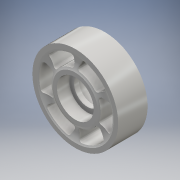
# Autodesk Inventor part: inner_wheel1
Saved by Autodesk Inventor 2016 (Build 200138000, 138)
## iProperties
Created: 2016-02-01
Part Number: inner_wheel1
Material: Aluminum 6061
Document SubType Name: Modeling
Designer: Carlo
Mass: 123.47 g
Surface Area: 198.887 cm^2
Volume: 45.7297 cm^3
Density: 2.7 g/cm^3
Appearance: Aluminum - Flat
Author: Carlo
Autodesk Inventor part; units mm, degrees
ref_plane "YZ Plane" through (0, 0, 0) normal (1, 0, 0) x (0, 1, 0)
ref_plane "XZ Plane" through (0, 0, 0) normal (0, 1, 0) x (-1, 0, 0)
ref_plane "XY Plane" through (0, 0, 0) normal (0, 0, 1) x (1, 0, 0)
sketch "Sketch1" plane through (0, 0, 0) normal (0, 1, 0) x (-1, 0, 0)
  circle A0 centre (0, 0) radius 35
  dimension "d0" = 70
  constraints: 1 centre point, 1 coincident
  measures "d0" diameter of A0
extrude "Extrusion1" add sketch "Sketch1" along normal mid plane 24
sketch "Sketch2" plane through (0, 12, 0) normal (0, 1, 0) x (1, 0, 0)
  line L0 (-24.5746, 17.2073) -> (-16.383, 11.4715)
  line L1 (-5.4819, 29.4949) -> (0, 20)
  arc A0 (-5.4819, 29.4949) -> (-24.5746, 17.2073) centre (0, 0) ccw
  arc A1 (0, 20) -> (-16.383, 11.4715) centre (0, 0) ccw
  line L2 (-16.383, 11.4715) -> (0, 0) construction
  line L3 (0, 0) -> (0, 35) construction
  circle A2 centre (0, 0) radius 35 construction
  dimension "d3" = 30
  dimension "d4" = 55
  dimension "d5" = 30
  dimension "d6" = 20
  constraints: 8 end point, 4 point on circle, 2 centre point, 1 collinear, 1 concentric, 1 point on line, 1 vertical, 1 vertical alignment, 2 other
  measures "d3" angle of L3 L1
  measures "d4" angle of L0 L3
  measures "d5" radius of A0
  measures "d6" radius of A1
extrude "Extrusion2" cut sketch "Sketch2" against normal through all
fillet "Fillet1" radius 2 4 edges at (-24.5746, 0, -17.2073) (-16.383, 0, -11.4715) (0, 0, -20) (-5.4819, 0, -29.4949)
pattern_circular "Circular Pattern1" count 6 over 360 about axis through (0, -10, 0) along (0, 1, 0) of "Extrusion2", "Fillet1"
hole "Hole1" at (0, 12, 0) direction (0, -1, 0) diameter 22 end through all
sketch "Sketch3" plane through (0, 12, 0) normal (0, 1, 0) x (1, 0, 0)
  point P0 (0, 0)
sketch "Sketch4" plane through (0, 12, 0) normal (0, 1, 0) x (1, 0, 0)
  point P0 (0, 0)
sketch "Sketch5" plane through (0, 12, 0) normal (0, 1, 0) x (1, 0, 0)
  circle A0 centre (0, 0) radius 15
  circle A1 centre (0, 0) radius 11 projected
  dimension "d22" = 30
  constraints: 1 centre point, 1 coincident, 1 concentric
  measures "d22" diameter of A0
extrude "Extrusion3" cut sketch "Sketch5" against normal blind 10
sketch "Sketch6" plane through (0, 0, 0) normal (0, 0, 1) x (1, 0, 0)
  line L0 (30, -12) -> (30, 12) projected
  line L1 (30, 12) -> (35, 12) projected
  line L2 (35, 12) -> (35, -12) projected
  line L3 (35, -12) -> (30, -12) projected
  line L4 (20, 12) -> (20, -12) projected
  line L5 (20, -12) -> (11, -12) projected
  line L6 (11, -12) -> (11, 2) projected
  line L7 (11, 2) -> (15, 2) projected
  line L8 (15, 2) -> (15, 12) projected
  line L9 (15, 12) -> (20, 12) projected
  line L10 (-30, 12) -> (-30, -12) projected
  line L11 (-30, -12) -> (-35, -12) projected
  line L12 (-35, -12) -> (-35, 12) projected
  line L13 (-35, 12) -> (-30, 12) projected
  line L14 (-20, -12) -> (-20, 12) projected
  line L15 (-20, 12) -> (-15, 12) projected
  line L16 (-15, 12) -> (-15, 2) projected
  line L17 (-15, 2) -> (-11, 2) projected
  line L18 (-11, 2) -> (-11, -12) projected
  line L19 (-11, -12) -> (-20, -12) projected
  line L20 (-35, -12) -> (35, -12) projected
  line L21 (-31.35, -12) -> (-18.3386, -12)
  line L22 (-4.7427, -12) -> (-21.7978, -12) projected
  arc A0 (-18.3386, -12) -> (-31.35, -12) centre (-24.8443, -25.5158) ccw
  line L23 (0, -33.0189) -> (0, 19.5032) projected
  point P0 (0, 0)
  dimension "d25" = 15
  constraints: 2 end point, 2 point on circle, 1 centre point, 1 point on line, 2 other
  measures "d25" radius of A0
revolve "Revolution1" cut sketch "Sketch6" angle 360 about axis through (0, -10, 0) along (0, 1, 0) contours L19 L14 A0 | L20 L10 A0 L14 | L10 L11 A0
mirror "Mirror1" about plane through (0, 0, 0) normal (0, 1, 0) of "Extrusion3", "Revolution1"
body "Solid1"
